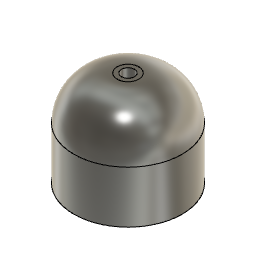
Porte_aimant_KOSMOS3-0 (Autodesk Fusion 360 design; units mm, degrees)
Autodesk Fusion 360 part; units mm, degrees
sketch "Esquisse1" plane through (0, 0, 0) normal (0, 0, 1) x (1, 0, 0)
  circle A0 centre (0, 0) radius 12.5
  line L0 (-5.3, -5.3) -> (5.3, -5.3)
  line L1 (5.3, -5.3) -> (5.3, 5.3)
  line L2 (5.3, 5.3) -> (-5.3, 5.3)
  line L3 (-5.3, 5.3) -> (-5.3, -5.3)
  dimension "d1" = 25
  dimension "d4" = 10.6
  dimension "d5" = 5.3
  dimension "d6" = 5.3
  constraint coincident A0.centre origin
  constraint horizontal L0
  constraint vertical L1
  constraint horizontal L2
  constraint vertical L3
  constraint equal L0 L3
  measures "d1" diameter of A0
  measures "d4" distance of L0.start L0.end
  measures "d5" distance of A0.centre L3
  measures "d6" distance of A0.centre L0
extrude "Extrusion1" add sketch "Esquisse1" along normal blind 22 contours A0 | L0 L1 L2 L3
extrude "Extrusion2" cut sketch "Esquisse1" along normal blind 6 contours L0 L1 L2 L3
sketch "Esquisse2" plane through (0, 0, 22) normal (0, 0, 1) x (-1, 0, 0)
  circle A0 centre (0, 0) radius 12.5
  circle A1 centre (0, 0) radius 1.5
  dimension "d9" = 3
  constraint coincident A0.centre A1.centre
  measures "d9" diameter of A1
extrude "Extrusion3" cut sketch "Esquisse2" against normal blind 22 contours A1
hole "Perçage2" at (0, 0, 6) direction (0, 0, 1) diameter 8 depth 10 tip angle 180
fillet "Congé1" radius 10 1 edges at (-11.6541, -4.5202, 22)
chamfer "Chanfrein1" distance 0.5 angle 45 4 edges at (-5.3, 0, 0) (0, -5.3, 0) (5.3, 0, 0) (0, 5.3, 0)
equation "d5 = d4 / 2"
equation "d6 = d5"
